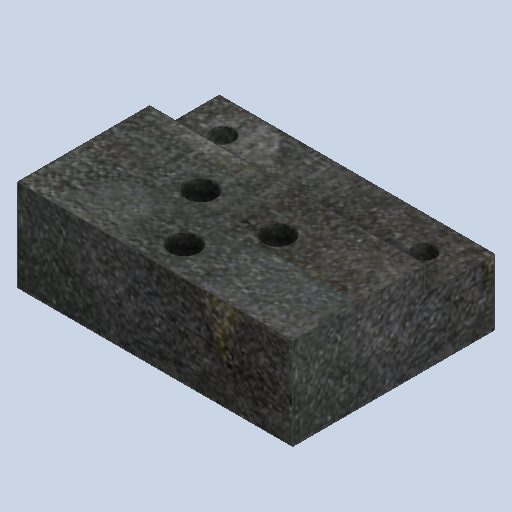
# Autodesk Inventor part: Feste Backe
Saved by Autodesk Inventor 2023.2 (Build 272271000, 271)
## iProperties
Created: 2023-02-05
Part Number: Feste Backe
Material: Steel
Document SubType Name: Modeling
Designer: Ayush
Density: 7.85 g/cm^3
Appearance: Plate
Author: Ayush
Autodesk Inventor part; units mm, degrees
ref_plane "YZ Plane" through (0, 0, 0) normal (1, 0, 0) x (0, 1, 0)
ref_plane "XZ Plane" through (0, 0, 0) normal (0, 1, 0) x (-1, 0, 0)
ref_plane "XY Plane" through (0, 0, 0) normal (0, 0, 1) x (1, 0, 0)
sketch "Sketch1" plane through (0, 0, 0) normal (0, 1, 0) x (-1, 0, 0)
  line L0 (-37.5, 27.5) -> (37.5, 27.5)
  line L1 (37.5, 27.5) -> (37.5, -27.5)
  line L2 (37.5, -27.5) -> (-37.5, -27.5)
  line L3 (-37.5, -27.5) -> (-37.5, 27.5)
  line L4 (-37.5, 27.5) -> (37.5, -27.5) construction
  line L5 (37.5, 27.5) -> (-37.5, -27.5) construction
  circle A0 centre (27.5, -18.5) radius 5.5
  circle A1 centre (-27.5, -18.5) radius 5.5
  circle A2 centre (0, 19.5) radius 7.5
  circle A3 centre (10.5, 4.5) radius 7.5
  circle A4 centre (-10.5, 4.5) radius 7.5
  point P0 (0, 0)
  point P1 (0, 27.5)
  dimension "d0" = 75
  dimension "d1" = 55
  dimension "d2" = 11
  dimension "d4" = 11
  dimension "d6" = 55
  dimension "d7" = 10
  dimension "d8" = 10
  dimension "d9" = 15
  dimension "d11" = 15
  dimension "d13" = 15
  dimension "d15" = 23
  dimension "d16" = 8
  dimension "d17" = 21
  dimension "d18" = 10.5
  dimension "d19" = 46
  constraints: 12 end point, 5 centre point, 3 midpoint, 2 parallel, 1 horizontal, 1 horizontal alignment, 1 perpendicular
  measures "d0" distance of L1.end L2.end
  measures "d1" distance of L0.end L1.end
  measures "d2" diameter of A0
  measures "d4" diameter of A1
  measures "d6" distance of A1.centre A0.centre
  measures "d7" distance from line of A0.centre L1
  measures "d8" distance from line of L3 A1.centre
  measures "d9" diameter of A2
  measures "d11" diameter of A3
  measures "d13" diameter of A4
  measures "d15" distance from line of A4.centre L0
  measures "d16" distance from line of A2.centre L0
  measures "d17" distance of A4.centre A3.centre
  measures "d18" horizontal distance of A4.centre point (0, 27.5)
  measures "d19" distance from line of L0 A0.centre
extrude "Extrusion1" add sketch "Sketch1" along normal blind 7
sketch "Sketch2" plane through (0, 7, 0) normal (0, 1, 0) x (1, 0, 0)
  line L0 (37.5, 27.5) -> (-37.5, 27.5) projected
  line L1 (37.5, -27.5) -> (-37.5, -27.5)
  line L2 (-37.5, -27.5) -> (-37.5, 27.5)
  line L3 (-37.5, 27.5) -> (37.5, 27.5)
  line L4 (37.5, 27.5) -> (37.5, -27.5)
  line L5 (37.5, -27.5) -> (-37.5, 27.5) construction
  line L6 (-37.5, -27.5) -> (37.5, 27.5) construction
  circle A0 centre (-27.5, 18.5) radius 3
  circle A1 centre (27.5, 18.5) radius 3
  circle A2 centre (-10.5, -4.5) radius 7.5
  circle A3 centre (10.5, -4.5) radius 7.5
  circle A4 centre (0, -19.5) radius 7.5
  circle A5 centre (0, -19.5) radius 4
  circle A6 centre (-10.5, -4.5) radius 4
  circle A7 centre (10.5, -4.5) radius 4
  line L7 (-37.5, -27.5) -> (37.5, -27.5) projected
  point P0 (0, 0)
  point P1 (0, -27.5)
  point P2 (0, -27.5)
  dimension "d22" = 6
  dimension "d23" = 6
  dimension "d24" = 15
  dimension "d25" = 15
  dimension "d26" = 15
  dimension "d27" = 8
  dimension "d28" = 8
  dimension "d29" = 8
  dimension "d30" = 55
  dimension "d31" = 10
  dimension "d32" = 10
  dimension "d33" = 46
  dimension "d34" = 23
  dimension "d35" = 8
  dimension "d36" = 10.5
  dimension "d37" = 10.5
  dimension "d38" = 21
  constraints: 12 end point, 8 centre point, 4 midpoint, 3 coincident, 2 parallel, 1 horizontal, 1 horizontal alignment, 1 perpendicular
  measures "d22" diameter of A0
  measures "d23" diameter of A1
  measures "d24" diameter of A2
  measures "d25" diameter of A3
  measures "d26" diameter of A4
  measures "d27" diameter of A5
  measures "d28" diameter of A6
  measures "d29" diameter of A7
  measures "d30" distance of A1.centre A0.centre
  measures "d31" distance from line of L2 A0.centre
  measures "d32" distance from line of L4 A1.centre
  measures "d33" distance from line of L1 A0.centre
  measures "d34" distance from line of A7.centre L1
  measures "d35" distance from line of L1 A4.centre
  measures "d36" horizontal distance of A3.centre point (0, -27.5)
  measures "d37" horizontal distance of point (0, -27.5) A2.centre
  measures "d38" distance of A3.centre A2.centre
extrude "Extrusion2" add sketch "Sketch2" along normal blind 3 contours L4 L1 L2 L0
sketch "Sketch3" plane through (0, 10, 0) normal (0, 1, 0) x (1, 0, 0)
  line L0 (37.5, 27.5) -> (-37.5, 27.5) projected
  line L1 (37.5, -27.5) -> (-37.5, -27.5)
  line L2 (-37.5, -27.5) -> (-37.5, 27.5)
  line L3 (-37.5, 27.5) -> (37.5, 27.5)
  line L4 (37.5, 27.5) -> (37.5, -27.5)
  line L5 (37.5, -27.5) -> (-37.5, 27.5) construction
  line L6 (-37.5, -27.5) -> (37.5, 27.5) construction
  circle A0 centre (-27.5, 18.5) radius 3 projected
  circle A1 centre (-27.5, 18.5) radius 3
  circle A2 centre (27.4955, 18.5) radius 3
  circle A3 centre (-10.5, -4.5) radius 4
  circle A4 centre (10.5, -4.5) radius 4
  circle A5 centre (0, -19.5) radius 4
  line L7 (-37.5, -27.5) -> (37.5, -27.5) projected
  point P0 (0, 0)
  point P1 (0, -27.5)
  point P2 (0, -27.5)
  dimension "d41" = 6
  dimension "d42" = 8
  dimension "d43" = 8
  dimension "d44" = 8
  dimension "d45" = 8
  dimension "d46" = 23
  dimension "d47" = 10.5
  dimension "d48" = 10.5
  constraints: 12 end point, 5 centre point, 4 midpoint, 2 parallel, 1 coincident, 1 horizontal, 1 horizontal alignment, 1 perpendicular
  measures "d41" diameter of A2
  measures "d42" diameter of A3
  measures "d43" diameter of A4
  measures "d44" diameter of A5
  measures "d45" distance from line of A5.centre L1
  measures "d46" distance from line of L1 A4.centre
  measures "d47" horizontal distance of point (0, -27.5) A4.centre
  measures "d48" horizontal distance of point (0, -27.5) A3.centre
extrude "Extrusion3" add sketch "Sketch3" along normal blind 8
sketch "Sketch4" plane through (0, 18, 0) normal (0, 1, 0) x (1, 0, 0)
  line L0 (-37.5, 8.5) -> (37.5, 8.5)
  line L1 (-37.5, -27.5) -> (37.5, -27.5) projected
  line L2 (-37.5, 27.5) -> (-37.5, -27.5) projected
  line L3 (-37.5, 8.5) -> (-37.5, -27.5)
  line L4 (-37.5, -27.5) -> (37.5, -27.5) projected
  line L5 (-37.5, -27.5) -> (37.5, -27.5)
  line L6 (37.5, -27.5) -> (37.5, 8.5)
  circle A0 centre (-10.5, -4.5) radius 4
  circle A1 centre (10.5, -4.5) radius 4
  circle A2 centre (0, -19.5) radius 4
  point P0 (0, 0)
  point P1 (0, -27.5)
  dimension "d51" = 75
  dimension "d52" = 36
  dimension "d53" = 8
  dimension "d54" = 8
  dimension "d55" = 8
  dimension "d56" = 8
  dimension "d57" = 23
  dimension "d58" = 21
  dimension "d59" = 10.5
  constraints: 8 end point, 3 centre point, 2 collinear, 1 horizontal, 1 horizontal alignment, 1 midpoint
  measures "d51" distance of L0.start L0.end
  measures "d52" distance between parallel lines of L0 L1
  measures "d53" diameter of A0
  measures "d54" diameter of A1
  measures "d55" diameter of A2
  measures "d56" distance from line of A2.centre L1
  measures "d57" distance from line of A1.centre L1
  measures "d58" distance of A0.centre A1.centre
  measures "d59" horizontal distance of point (0, -27.5) A1.centre
extrude "Extrusion4" add sketch "Sketch4" along normal blind 7
body "Solid1"
